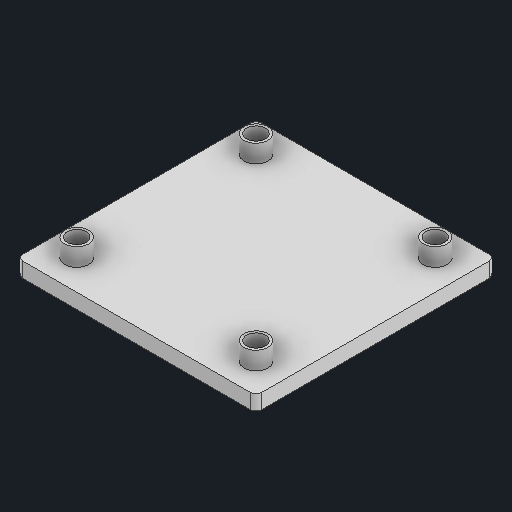
# Autodesk Inventor part: cradle_top
Saved by Autodesk Inventor 2025 (Build 290162010, 162A)
## iProperties
Created: 2024-06-21
Part Number: cradle_top
Material: Generic
Document SubType Name: Modeling
Designer: mihir
Density: 1 g/cm^3
Appearance: Default
Author: mihir
Autodesk Inventor part; units mm, degrees
ref_plane "YZ Plane" through (0, 0, 0) normal (1, 0, 0) x (0, 1, 0)
ref_plane "XZ Plane" through (0, 0, 0) normal (0, 1, 0) x (-1, 0, 0)
ref_plane "XY Plane" through (0, 0, 0) normal (0, 0, 1) x (1, 0, 0)
sketch "Sketch1" plane through (0, 0, 0) normal (0, 1, 0) x (-1, 0, 0)
  line L0 (0, 0) -> (80, 0)
  line L1 (80, 0) -> (80, -80)
  line L2 (80, -80) -> (0, -80)
  line L3 (0, -80) -> (0, 0)
  dimension "d0" = 80
  constraints: 8 end point, 2 parallel, 2 perpendicular, 1 horizontal
  measures "d0" distance of L0.end L1.end
extrude "Extrusion1" add sketch "Sketch1" along normal blind 5
fillet "Fillet1" radius 2 4 edges at (-80, 2.5, 0) (-80, 2.5, -80) (0, 2.5, -80) (0, 2.5, 0)
sketch "Sketch2" plane through (0, 5, 0) normal (0, 1, 0) x (1, 0, 0)
  line L0 (-10, 10) -> (-70, 10) construction
  line L1 (-70, 10) -> (-70, 70) construction
  line L2 (-70, 70) -> (-10, 70) construction
  line L3 (-10, 70) -> (-10, 10) construction
  line L4 (0, 2) -> (0, 78) construction
  line L5 (-78, 0) -> (-2, 0) construction
  circle A0 centre (-70, 10) radius 3.15
  circle A1 centre (-70, 70) radius 3.15
  circle A2 centre (-10, 70) radius 3.15
  circle A3 centre (-10, 10) radius 3.15
  circle A4 centre (-70, 10) radius 4
  circle A5 centre (-70, 70) radius 4
  circle A6 centre (-10, 70) radius 4
  circle A7 centre (-10, 10) radius 4
  point P0 (0, 0)
  dimension "d4" = 60
  dimension "d5" = 10
  dimension "d6" = 10
  dimension "d7" = 6.3
  dimension "d8" = 8
  constraints: 8 centre point, 8 coincident, 8 end point, 6 equal radius, 3 perpendicular, 1 horizontal, 1 vertical
  measures "d4" distance of L0.end L1.end
  measures "d5" distance from line of L4 L0.start
  measures "d6" distance from line of L5 L0.start
  measures "d7" diameter of A0
  measures "d8" diameter of A4
extrude "Extrusion2" add sketch "Sketch2" along normal blind 6
equation "\"d0\" = cradle_width"
equation "\"d4\" = rod_dist"
equation "\"d5\" = 0.5 * cradle_width - 0.5 * rod_dist"
equation "\"d6\" = 0.5 * cradle_width - 0.5 * rod_dist"
equation "\"d7\" = rod_diameter + rod_tolerance"
equation "\"d8\" = post_diameter"
equation "\"cradle_width\" = 80"
equation "\"rod_diameter\" = 6"
equation "\"rod_tolerance\" = 0.3"
equation "\"post_diameter\" = 8"
equation "\"rod_dist\" = 60"
body "Solid1"
